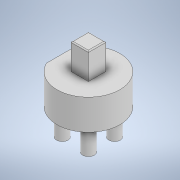
# Autodesk Inventor part: D6L90 F1 LFS
Saved by Autodesk Inventor 2021 (Build 250183000, 183)
## iProperties
Created: 2021-03-23
Part Number: D6L90 F1 LFS
Material: Generic
Document SubType Name: Modeling
Designer: ben
Density: 1 g/cm^3
Appearance: Default
Author: ben
Autodesk Inventor part; units mm, degrees
ref_plane "YZ Plane" through (0, 0, 0) normal (1, 0, 0) x (0, 1, 0)
ref_plane "XZ Plane" through (0, 0, 0) normal (0, 1, 0) x (-1, 0, 0)
ref_plane "XY Plane" through (0, 0, 0) normal (0, 0, 1) x (1, 0, 0)
sketch "Sketch1" plane through (0, 0, 0) normal (0, 1, 0) x (-1, 0, 0)
  arc A0 (5.4, 2.6153) -> (5.4, -2.6153) centre (0, 0) ccw
  line L0 (1.65, 1.65) -> (-1.65, 1.65)
  line L1 (-1.65, 1.65) -> (-1.65, -1.65)
  line L2 (-1.65, -1.65) -> (1.65, -1.65)
  line L3 (1.65, -1.65) -> (1.65, 1.65)
  line L4 (1.65, 1.65) -> (-1.65, -1.65) construction
  line L5 (-1.65, 1.65) -> (1.65, -1.65) construction
  line L6 (5.4, -2.6153) -> (5.4, 2.6153)
  circle A1 centre (2.5, 2.5) radius 1.1
  circle A2 centre (2.5, -2.5) radius 1.1
  circle A3 centre (-2.5, 2.5) radius 1.1
  circle A4 centre (-2.5, -2.5) radius 1.1
  point P0 (-6, 0)
  dimension "d0" = 12
  dimension "d1" = 3.3
  dimension "d2" = 3.3
  dimension "d3" = 11.4
  dimension "d4" = 2.2
  dimension "d7" = 5
  dimension "d10" = 5
  constraints: 14 end point, 5 centre point, 3 point on circle, 3 vertical, 2 horizontal, 2 midpoint, 2 parallel, 1 coincident, 1 perpendicular, 7 other
  measures "d0" diameter of A0
  measures "d1" distance of L2.end L1.end
  measures "d2" distance of L1.end L0.end
  measures "d3" distance from line of L6 point (-6, 0)
  measures "d4" diameter of A1
  measures "d7" distance of A1.centre A2.centre
  measures "d10" distance of A1.centre A3.centre
extrude "Extrusion1" add sketch "Sketch1" along normal blind 5.8 contours L6 A0 | A1 | A2 | A3 | A4
extrude "Extrusion2" add sketch "Sketch1" along normal blind 10.8 contours L3 L2 L1 L0
extrude "Extrusion3" add sketch "Sketch1" against normal blind 5 contours A1 | A2 | A3 | A4
fillet "Fillet1" radius 0.2 4 edges at (0, 10.8, -1.65) (-1.65, 10.8, 0) (0, 10.8, 1.65) (1.65, 10.8, 0)
body "Solid1"
